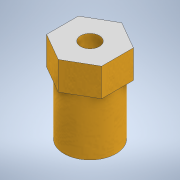
# Autodesk Inventor part: Coupling
Saved by Autodesk Inventor 2022 (Build 260153000, 153)
## iProperties
Created: 2023-03-17
Part Number: Coupling
Material: 一般
Document SubType Name: Modeling
Designer: JOU
Density: 1 g/cm^3
Appearance: 預設
Mass: 1.64153 g
Surface Area: 11.3377 cm^2
Volume: 1.64153 cm^3
Author: JOU
Autodesk Inventor part; units mm, degrees
ref_plane "XZ Plane" through (0, 0, 0) normal (0, 1, 0) x (-1, 0, 0)
ref_plane "XY Plane" through (0, 0, 0) normal (0, 0, 1) x (1, 0, 0)
sketch "草圖1" plane through (0, 0, 0) normal (0, 1, 0) x (-1, 0, 0)
  circle A0 centre (0, 0) radius 5.5
  dimension "d0" = 11
  constraints: 1 centre point, 1 coincident
  measures "d0" diameter of A0
extrude "擠出1" add sketch "草圖1" along normal blind 12
sketch "草圖2" plane through (0, 12, 0) normal (0, 1, 0) x (1, 0, 0)
  line L0 (5.85, -3.3775) -> (0, -6.755)
  line L1 (0, -6.755) -> (-5.85, -3.3775)
  line L2 (-5.85, -3.3775) -> (-5.85, 3.3775)
  line L3 (-5.85, 3.3775) -> (0, 6.755)
  line L4 (0, 6.755) -> (5.85, 3.3775)
  line L5 (5.85, 3.3775) -> (5.85, -3.3775)
  point P0 (0, 0)
  point P1 (0, 0)
  dimension "d3" = 11.7
  constraints: 12 end point, 1 coincident, 1 vertical, 13 other
  measures "d3" distance between parallel lines of L5 L2
extrude "擠出2" add sketch "草圖2" along normal blind 6
sketch "草圖3" plane through (0, 0, 0) normal (0, -1, 0) x (1, 0, 0)
  circle A0 centre (0, 0) radius 2
  dimension "d6" = 4
  constraints: 1 centre point, 1 coincident
  measures "d6" diameter of A0
extrude "擠出3" cut sketch "草圖3" against normal up to surface (18 mm away)
sketch "草圖5" plane through (0, 0, 0) normal (1, 0, 0) x (0, 1, 0)
  circle A0 centre (4, 0) radius 1.361
  point P0 (0, 0)
  dimension "d12" = 4
  constraints: 1 centre point, 1 horizontal alignment
  measures "d12" distance of point (0, 0) A0.centre
extrude "擠出5" cut sketch "草圖5" against normal through all
sketch "草圖6" plane through (0, 0, 0) normal (0, -1, 0) x (1, 0, 0)
  circle A0 centre (0, 0) radius 2 projected
  circle A1 centre (0, 0) radius 5.5 projected
  circle A2 centre (0, 0) radius 2 projected
  line L0 (1.0536, 1.7) -> (-1.0536, 1.7)
  dimension "d15" = 1.7
  constraints: 2 end point, 2 point on circle, 1 horizontal
  measures "d15" distance from line of L0 point (0, 0)
ref_plane "工作平面2" through (-5.5, 0, 0) normal (1, 0, 0) x (0, 1, 0)
ref_plane "工作平面1" through (5.5, 0, 0) normal (1, 0, 0) x (0, 1, 0)
sketch "草圖7" plane through (-5.5, 0, 0) normal (1, 0, 0) x (0, 1, 0)
  spline S0 degree 5 poles (5.361, 0) (5.361, 0.1236) (5.347, 0.2463) (5.3194, 0.3649) (5.2798, 0.4768) (5.1704, 0.7094) (5.0945, 0.8261) (5.0077, 0.929) (4.9122, 1.0182) (4.67, 1.1972) (4.517, 1.2762) (4.3518, 1.3325) (4.1759, 1.361) (3.8245, 1.361) (3.6486, 1.3326) (3.4837, 1.2765) (3.3306, 1.1975) (3.1182, 1.0408) (3.0486, 0.98) (2.9834, 0.9125) (2.9233, 0.8382) (2.7861, 0.6333) (2.7171, 0.4936) (2.6652, 0.3374) (2.639, 0.1686) (2.639, -0.1236) (2.653, -0.2463) (2.6806, -0.3649) (2.7202, -0.4768) (2.8296, -0.7094) (2.9055, -0.8261) (2.9923, -0.929) (3.0878, -1.0182) (3.33, -1.1972) (3.483, -1.2762) (3.6482, -1.3325) (3.8241, -1.361) (4.1755, -1.361) (4.3514, -1.3326) (4.5163, -1.2765) (4.6694, -1.1975) (4.9141, -1.0169) (5.0116, -0.9254) (5.1001, -0.8195) (5.177, -0.6991) (5.2842, -0.4643) (5.3217, -0.355) (5.3478, -0.2394) (5.361, -0.1201) (5.361, 0) knots 0 0 0 0 0 0 0.063036 0.063036 0.063036 0.063036 0.142762 0.142762 0.142762 0.142762 0.249982 0.249982 0.249982 0.249982 0.35698 0.35698 0.35698 0.35698 0.413527 0.413527 0.413527 0.413527 0.499667 0.499667 0.499667 0.499667 0.562796 0.562796 0.562796 0.562796 0.64264 0.64264 0.64264 0.64264 0.750018 0.750018 0.750018 0.750018 0.857175 0.857175 0.857175 0.857175 0.93874 0.93874 0.93874 0.93874 1 1 1 1 1 1 projected
  circle A0 centre (4, 0) radius 1.5
  point P0 (0, 0)
  dimension "d17" = 3
  constraints: 1 centre point, 1 other
  measures "d17" diameter of A0
extrude "擠出6" cut sketch "草圖7" along normal blind 1.5
